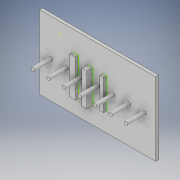
# Autodesk Inventor part: gearbasephonecaseFINAL
Saved by Autodesk Inventor 2018 (Build 220112000, 112)
## iProperties
Created: 2019-03-18
Part Number: gearbasephonecaseFINAL
Material: Generic
Document SubType Name: Modeling
Designer: F8PLTW
Density: 1 g/cm^3
Appearance: Default
Author: F8PLTW
Autodesk Inventor part; units mm, degrees
ref_plane "YZ Plane" through (0, 0, 0) normal (1, 0, 0) x (0, 1, 0)
ref_plane "XZ Plane" through (0, 0, 0) normal (0, 1, 0) x (-1, 0, 0)
ref_plane "XY Plane" through (0, 0, 0) normal (0, 0, 1) x (1, 0, 0)
sketch "Sketch1" plane through (0, 0, 0) normal (0, 0, 1) x (1, 0, 0)
  line L0 (-22.1112, 10.3171) -> (130.2888, 10.3171)
  line L1 (130.2888, 10.3171) -> (130.2888, -65.8829)
  line L2 (130.2888, -65.8829) -> (-22.1112, -65.8829)
  line L3 (-22.1112, -65.8829) -> (-22.1112, 10.3171)
  point P0 (0, 0)
  dimension "d0" = 152.4
  dimension "d1" = 76.2
  constraints: 8 end point, 2 parallel, 1 horizontal, 1 perpendicular
  measures "d0" distance of L1.end L2.end
  measures "d1" distance of L0.end L1.end
extrude "Extrusion1" add sketch "Sketch1" along normal blind 3.175
sketch "Sketch2" plane through (0, 0, 3.175) normal (0, 0, 1) x (1, 0, 0)
  circle A0 centre (-10.0607, -27.9271) radius 1.85
  circle A1 centre (6.0853, -27.9271) radius 1.85
  circle A2 centre (22.2313, -27.9271) radius 1.85
  circle A3 centre (38.3773, -27.9271) radius 1.85
  circle A4 centre (54.5233, -27.9271) radius 1.85
  circle A5 centre (70.6693, -27.9271) radius 1.85
  circle A6 centre (86.8153, -27.9271) radius 1.85
  point P0 (0, 0)
  dimension "d4" = 3.7
  dimension "d5" = 3.7
  dimension "d6" = 3.7
  dimension "d7" = 12.446
  dimension "d8" = 12.446
  dimension "d9" = 3.7
  dimension "d10" = 12.446
  dimension "d11" = 3.7
  dimension "d12" = 3.7
  dimension "d13" = 3.7
  dimension "d14" = 12.446
  dimension "d15" = 12.446
  dimension "d16" = 12.446
  constraints: 7 centre point
  measures "d4" diameter of A0
  measures "d5" diameter of A1
  measures "d6" diameter of A2
  measures "d9" diameter of A3
  measures "d11" diameter of A4
  measures "d12" diameter of A5
  measures "d13" diameter of A6
extrude "Extrusion2" add sketch "Sketch2" along normal blind 19.05
sketch "Sketch3" plane through (130.2888, -65.8829, 0) normal (1, 0, 0) x (0, 0, -1)
  line L0 (-11.1509, 83.1688) -> (7.2167, 83.1688)
  line L1 (7.2167, 83.1688) -> (7.2167, -5.5026)
  line L2 (7.2167, -5.5026) -> (-11.1509, -5.5026)
  line L3 (-11.1509, -5.5026) -> (-11.1509, 83.1688)
  point P0 (0, 65.8829)
  constraints: 8 end point, 2 parallel, 1 horizontal, 1 perpendicular
extrude "Extrusion3" cut sketch "Sketch3" against normal blind 31.75
sketch "Sketch4" plane through (0, 0, 3.175) normal (0, 0, 1) x (1, 0, 0)
  line L0 (43.7795, -14.066) -> (47.6081, -14.066)
  line L1 (47.6081, -14.066) -> (47.6081, -46.0267)
  line L2 (47.6081, -46.0267) -> (43.7795, -46.0267)
  line L3 (43.7795, -46.0267) -> (43.7795, -14.066)
  line L4 (33.3021, -14.066) -> (28.2479, -14.066)
  line L5 (28.2479, -14.066) -> (28.2479, -48.0243)
  line L6 (28.2479, -48.0243) -> (33.3021, -48.0243)
  line L7 (33.3021, -48.0243) -> (33.3021, -14.066)
  line L8 (12.2443, -10.6645) -> (18.3845, -10.6645)
  line L9 (18.3845, -10.6645) -> (18.3845, -49.2753)
  line L10 (18.3845, -49.2753) -> (12.2443, -49.2753)
  line L11 (12.2443, -49.2753) -> (12.2443, -10.6645)
  point P0 (0, 0)
  constraints: 24 end point, 6 parallel, 3 horizontal, 3 perpendicular
extrude "Extrusion4" [suppressed]
extrude "Extrusion5" [suppressed]
extrude "Extrusion6" add sketch "Sketch4" along normal blind 3.175 contours L0 L1 L2 L3 | L8 L9 L10 L11
extrude "Extrusion7" add sketch "Sketch4" along normal blind 6.35 contours L7 L6 L5 L4
body "Solid1"
